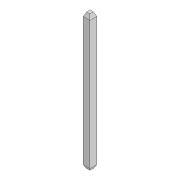
# Autodesk Inventor part: Molex_0901_pin
Saved by Autodesk Inventor 2021 (Build 250183000, 183)
## iProperties
Created: 2021-10-07
Part Number: Molex_0901_pin
Material: Generic
Document SubType Name: Modeling
Designer: WSE-PC04
Density: 1 g/cm^3
Appearance: Default
Author: WSE-PC04
Autodesk Inventor part; units mm, degrees
ref_plane "YZ Plane" through (0, 0, 0) normal (1, 0, 0) x (0, 1, 0)
ref_plane "XZ Plane" through (0, 0, 0) normal (0, 1, 0) x (-1, 0, 0)
ref_plane "XY Plane" through (0, 0, 0) normal (0, 0, 1) x (1, 0, 0)
sketch "Sketch1" plane through (0, 0, 0) normal (0, 1, 0) x (-1, 0, 0)
  line L0 (0.33, 0.33) -> (-0.33, 0.33)
  line L1 (-0.33, 0.33) -> (-0.33, -0.33)
  line L2 (-0.33, -0.33) -> (0.33, -0.33)
  line L3 (0.33, -0.33) -> (0.33, 0.33)
  line L4 (0.33, 0.33) -> (-0.33, -0.33) construction
  line L5 (-0.33, 0.33) -> (0.33, -0.33) construction
  point P0 (0, 0)
  dimension "d0" = 0.66
  dimension "d1" = 0.66
  constraints: 12 end point, 2 midpoint, 2 parallel, 1 horizontal, 1 perpendicular
  measures "d0" distance of L1.end L2.end
  measures "d1" distance of L0.end L1.end
extrude "Extrusion1" add sketch "Sketch1" along normal blind 4.64 and the other way blind 8.4
chamfer "Chamfer13" distance 0.17 distance2 0.38 1 edges at (0.33, 4.64, 0) measured on face at (0.11, 4.64, 0.11)
chamfer "Chamfer14" distance 0.17 distance2 0.38 1 edges at (-0.33, 4.64, 0) measured on face at (-0.0033, 4.64, 0.11)
chamfer "Chamfer15" distance 0.17 distance2 0.38 1 edges at (0, 4.64, 0.33) measured on face at (0.0533, 4.64, 0.11)
chamfer "Chamfer16" distance 0.17 distance2 0.38 1 edges at (0, 4.64, -0.33) measured on face at (0.0533, 4.64, -0.0033)
chamfer "Chamfer17" distance 0.15 distance2 0.3 1 edges at (0.33, -8.4, 0) measured on face at (0.11, -8.4, 0.11)
chamfer "Chamfer18" distance 0.15 distance2 0.3 1 edges at (-0.33, -8.4, 0) measured on face at (0.01, -8.4, 0.11)
chamfer "Chamfer19" distance 0.15 distance2 0.3 1 edges at (0, -8.4, 0.33) measured on face at (0.06, -8.4, 0.11)
chamfer "Chamfer20" distance 0.15 distance2 0.3 1 edges at (0, -8.4, -0.33) measured on face at (0.06, -8.4, 0.01)
body "Solid1"
